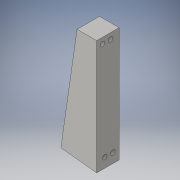
# Autodesk Inventor part: Ball screw support [bed]
Saved by Autodesk Inventor 2016 (Build 200138000, 138)
## iProperties
Created: 2017-05-16
Part Number: Ball screw support [bed]
Material: Generic
Document SubType Name: Modeling
Designer: m228540
Density: 1 g/cm^3
Appearance: Default
Author: m228540
Autodesk Inventor part; units mm, degrees
ref_plane "YZ Plane" through (0, 0, 0) normal (1, 0, 0) x (0, 1, 0)
ref_plane "XZ Plane" through (0, 0, 0) normal (0, 1, 0) x (-1, 0, 0)
ref_plane "XY Plane" through (0, 0, 0) normal (0, 0, 1) x (1, 0, 0)
sketch "Sketch1" plane through (0, 0, 0) normal (0, 0, 1) x (1, 0, 0)
  line L0 (9.4247, 103.8012) -> (9.4247, -95.1988)
  line L1 (9.4247, -95.1988) -> (-52.5753, -88.1988)
  line L2 (-52.5753, -88.1988) -> (-24.5753, 103.8012)
  line L3 (-24.5753, 103.8012) -> (9.4247, 103.8012)
  point P0 (0, 0)
  dimension "d0" = 199
  dimension "d1" = 62
  dimension "d2" = 34
  dimension "d3" = 7
  constraints: 8 end point, 1 perpendicular, 1 vertical
  measures "d0" distance of L0.start L0.end
  measures "d1" distance from line of L0 L1.end
  measures "d2" distance of L2.end L0.start
  measures "d3" vertical distance of L0.end L1.end
extrude "Extrusion1" add sketch "Sketch1" along normal blind 39
sketch "Sketch2" plane through (9.4247, -95.1988, 0) normal (1, 0, 0) x (0, 0, -1)
  circle A0 centre (-11, 17) radius 4
  circle A1 centre (-25, 17) radius 4
  circle A2 centre (-15, 189) radius 4
  circle A3 centre (-29, 189) radius 4
  line L0 (-39, 0) -> (-39, 199) projected
  line L1 (0, 0) -> (-39, 0) projected
  line L2 (0, 199) -> (-39, 199) projected
  point P0 (0, 95.1988)
  dimension "d6" = 8
  dimension "d7" = 8
  dimension "d8" = 14
  dimension "d9" = 14
  dimension "d10" = 172
  dimension "d11" = 8
  dimension "d12" = 8
  dimension "d13" = 14
  dimension "d14" = 10
  dimension "d18" = 10
  constraints: 4 centre point, 2 horizontal alignment
  measures "d6" diameter of A0
  measures "d7" diameter of A1
  measures "d8" distance from line of L0 A1.centre
  measures "d9" distance of A0.centre A1.centre
  measures "d10" vertical distance of A0.centre A2.centre
  measures "d11" diameter of A2
  measures "d12" diameter of A3
  measures "d13" distance of A2.centre A3.centre
  measures "d14" distance from line of L0 A3.centre
  measures "d18" distance from line of L2 A2.centre
extrude "Extrusion2" cut sketch "Sketch2" against normal through all
body "Solid1"
